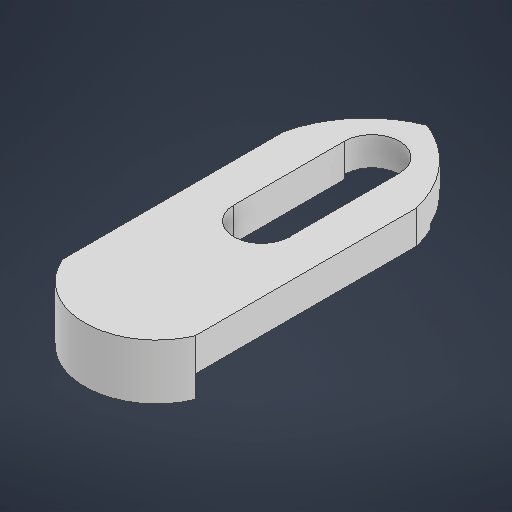
# Autodesk Inventor part: Carrier Tab
Saved by Autodesk Inventor 2026.2 (Build 302298010, 298A)
## iProperties
Created: 2026-04-23
Part Number: Carrier Tab
Material: Generic
Document SubType Name: Modeling
Designer: cfang
Density: 1 g/cm^3
Appearance: Default
Author: cfang
Autodesk Inventor part; units mm, degrees
ref_plane "YZ Plane" through (0, 0, 0) normal (1, 0, 0) x (0, 1, 0)
ref_plane "XZ Plane" through (0, 0, 0) normal (0, 1, 0) x (-1, 0, 0)
ref_plane "XY Plane" through (0, 0, 0) normal (0, 0, 1) x (1, 0, 0)
sketch "Sketch1" plane through (0, 0, 0) normal (0, 1, 0) x (-1, 0, 0)
  line L0 (-3, -8) -> (3, -8)
  line L1 (3, -8) -> (3, 8)
  line L2 (3, 8) -> (-3, 8)
  line L3 (-3, 8) -> (-3, -8)
  line L4 (-3, -8) -> (3, 8) construction
  line L5 (3, -8) -> (-3, 8) construction
  point P0 (0, 0)
  dimension "d0" = 16
  dimension "d1" = 6
  constraints: 12 end point, 2 midpoint, 2 parallel, 1 horizontal, 1 perpendicular
  measures "d0" distance of L0.end L1.end
  measures "d1" distance of L1.end L2.end
extrude "Extrusion1" add sketch "Sketch1" along normal blind 2.5
sketch "Sketch2" plane through (0, 2.5, 0) normal (0, 1, 0) x (1, 0, 0)
  line L0 (0, 5) -> (0, 0) construction
  line L1 (-1.25, 5) -> (-1.25, 0)
  line L2 (1.25, 0) -> (1.25, 5)
  arc A0 (1.25, 5) -> (-1.25, 5) centre (0, 5) ccw
  arc A1 (-1.25, 0) -> (1.25, 0) centre (0, 0) ccw
  line L3 (-3, -8) -> (3, -8) projected
  line L4 (-3, 8) -> (-3, -8) projected
  line L5 (-3, -8) -> (3, -8) projected
  line L6 (3, -8) -> (3, 8) projected
  line L7 (3, 8) -> (-3, 8) projected
  point P0 (0, 2.5)
  point P1 (0, 2.5)
  dimension "d4" = 2.5
  dimension "d6" = 8
  dimension "d7" = 6
  dimension "d8" = 3
  dimension "d9" = 5
  constraints: 8 end point, 4 point on circle, 4 tangent, 2 centre point, 1 coincident, 1 midpoint, 1 parallel, 1 vertical
  measures "d4" distance between parallel lines of L1 L2
  measures "d6" distance from line of L3 L0.end
  measures "d7" distance of L3.start L3.end
  measures "d8" distance from line of L4 point (0, 2.5)
  measures "d9" distance of L0.end L0.start
extrude "Extrusion2" cut sketch "Sketch2" against normal through all contours A0 L2 A1 L1
sketch "Sketch3" plane through (3, 0, 8) normal (1, 0, 0) x (0, 0, -1)
  line L0 (16, 0) -> (0, 0) projected
  line L1 (16, 0) -> (2, 0)
  line L2 (2, 0) -> (2, 1)
  line L3 (2, 1) -> (16, 1)
  line L4 (16, 1) -> (16, 0)
  line L5 (0, 0) -> (0, 2.5) projected
  line L6 (0, 2.5) -> (16, 2.5) projected
  point P0 (8, 0)
  point P1 (2, 0)
  dimension "d12" = 2
  dimension "d13" = 1.5
  constraints: 8 end point, 2 parallel, 1 horizontal, 1 perpendicular
  measures "d12" distance between parallel lines of L2 L5
  measures "d13" distance between parallel lines of L6 L3
extrude "Extrusion3" cut sketch "Sketch3" against normal through all
sketch "Sketch4" plane through (0, 2.5, 0) normal (0, 1, 0) x (1, 0, 0)
  line L0 (-3, 8) -> (-3, -8) projected
  line L1 (3, -8) -> (3, 8) projected
  arc A0 (-3, -6) -> (3, -6) centre (0, -4.75) ccw
  line L2 (-3, -8) -> (3, -8) projected
  point P0 (0, 0)
  point P1 (-2, 6)
  point P2 (2, 6)
  point P3 (3, 8)
  point P4 (0, -8)
  point P5 (-2.2361, -8)
  dimension "d17" = 2
  constraints: 2 point on circle, 1 centre point, 1 horizontal alignment, 1 tangent, 4 other
  measures "d17" distance from line of L2 A0.start
extrude "Extrusion4" cut sketch "Sketch4" against normal through all
sketch "Sketch5" plane through (0, 2.5, 0) normal (0, 1, 0) x (1, 0, 0)
  line L0 (3, -6) -> (3, 8) projected
  line L1 (3, 8) -> (-3, 8) projected
  line L2 (-3, 8) -> (-3, -6) projected
  arc A0 (1.25, 5) -> (-1.25, 5) centre (0, 5) ccw projected
  arc A1 (3, 4) -> (0, 7.5) centre (-1.8689, 2.8624) ccw
  arc A2 (0, 7.5) -> (-3, 4) centre (1.8689, 2.8624) ccw
  point P0 (0, 0)
  point P1 (-3, 6.2041)
  point P2 (0, 6.25)
  point P3 (0, 6.25)
  dimension "d23" = 5
  dimension "d24" = 4
  dimension "d25" = 0.5
  constraints: 6 point on circle, 3 point on line, 2 centre point, 1 equal radius, 1 vertical alignment
  measures "d23" radius of A1
  measures "d24" distance from line of L1 A1.start
  measures "d25" distance from line of A1.end L1
extrude "Extrusion5" cut sketch "Sketch5" against normal through all
sketch "Sketch6" plane through (-3, 1, 6) normal (0, -1, 0) x (1, 0, 0)
  line L0 (6.1469, -11) -> (-0.0299, -11)
  line L1 (-0.0299, -11) -> (-0.0299, -13.5)
  line L2 (-0.0299, -13.5) -> (6.1469, -13.5)
  line L3 (6.1469, -13.5) -> (6.1469, -11)
  arc A0 (1.75, -11) -> (4.25, -11) centre (3, -11) ccw projected
  point P0 (3, -6)
  point P1 (3, -13.5)
  point P2 (1.75, -11)
  constraints: 8 end point, 2 parallel, 2 point on line, 1 horizontal, 1 perpendicular
extrude "Extrusion6" cut sketch "Sketch6" against normal blind 0.2 contours L3 L2 L1 L0 A0
equation "\"d8\" = 0.5 * d7"
body "Solid1"
